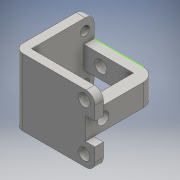
# Autodesk Inventor part: 240510_3Dsketch04
Saved by Autodesk Inventor 2016 (Build 200138000, 138)
## iProperties
Created: 2024-05-10
Part Number: 240510_3Dsketch04
Material: 일반
Document SubType Name: Modeling
Designer: pc
Density: 1 g/cm^3
Appearance: 기본값
Author: pc
Autodesk Inventor part; units mm, degrees
ref_plane "YZ Plane" through (0, 0, 0) normal (1, 0, 0) x (0, 1, 0)
ref_plane "XZ Plane" through (0, 0, 0) normal (0, 1, 0) x (-1, 0, 0)
ref_plane "XY Plane" through (0, 0, 0) normal (0, 0, 1) x (1, 0, 0)
sketch "스케치1" plane through (0, 0, 0) normal (0, 0, 1) x (1, 0, 0)
  line L0 (18.1059, -15.875) -> (-18.1059, -15.875)
  line L1 (-18.1059, -15.875) -> (-18.1059, 15.875)
  line L2 (-18.1059, 15.875) -> (18.1059, 15.875)
  line L3 (18.1059, 15.875) -> (18.1059, -15.875)
  line L4 (18.1059, -15.875) -> (-18.1059, 15.875) construction
  line L5 (-18.1059, -15.875) -> (18.1059, 15.875) construction
  point P0 (0, 0)
  constraints: 12 end point, 2 midpoint, 2 parallel, 1 horizontal, 1 perpendicular
extrude "돌출1" add sketch "스케치1" along normal blind 30
sketch "스케치2" plane through (-18.1059, 15.875, 0) normal (0, 1, 0) x (1, 0, 0)
  line L0 (0, -30) -> (36.2119, -30) projected
  line L1 (36.2119, 0) -> (36.2119, -30) projected
  line L2 (4.0585, -30) -> (36.2119, -30)
  line L3 (36.2119, -30) -> (36.2119, -19.9659)
  line L4 (36.2119, -19.9659) -> (4.0585, -19.9659)
  line L5 (4.0585, -19.9659) -> (4.0585, -30)
  line L6 (36.2119, 0) -> (0, 0) projected
  line L7 (4.0585, 0) -> (36.2119, 0)
  line L8 (36.2119, 0) -> (36.2119, -10.034)
  line L9 (36.2119, -10.034) -> (4.0585, -10.034)
  line L10 (4.0585, -10.034) -> (4.0585, 0)
  point P0 (18.1059, 0)
  dimension "d2" = 10.034
  constraints: 16 end point, 5 point on line, 4 parallel, 2 horizontal, 2 perpendicular
  measures "d2" distance of L7.end L8.end
extrude "돌출2" cut sketch "스케치2" against normal blind 28
sketch "스케치3" plane through (-18.1059, 15.875, 30) normal (0, 1, 0) x (1, 0, 0)
  line L0 (4.0585, 10.0341) -> (36.2119, 10.0341) projected
  line L1 (36.2119, 30) -> (36.2119, 0) projected
  line L2 (31.9669, 10.0341) -> (36.2119, 10.0341)
  line L3 (36.2119, 10.0341) -> (36.2119, 20.0064)
  line L4 (36.2119, 20.0064) -> (31.9669, 20.0064)
  line L5 (31.9669, 20.0064) -> (31.9669, 10.0341)
  point P0 (18.1059, 30)
  constraints: 8 end point, 2 parallel, 2 point on line, 1 horizontal, 1 perpendicular
extrude "돌출3" cut sketch "스케치3" against normal blind 50
sketch "스케치4" plane through (-14.0475, -12.125, 19.9659) normal (0, 0, 1) x (1, 0, 0)
  line L0 (0, 0) -> (22.1415, 0)
  line L1 (22.1415, 0) -> (22.1415, 23.4499)
  line L2 (22.1415, 23.4499) -> (0, 23.4499)
  line L3 (0, 23.4499) -> (0, 0)
  point P0 (14.0475, 12.125)
  constraints: 8 end point, 2 parallel, 1 horizontal, 1 perpendicular
extrude "돌출4" cut sketch "스케치4" against normal blind 50
sketch "스케치5" plane through (-14.0475, 15.875, 30) normal (1, 0, 0) x (0, 0, -1)
  circle A0 centre (5.0001, -4.0724) radius 2.0226
  circle A1 centre (25.7482, -4.0724) radius 2.1705
  point P0 (30, -15.875)
  constraints: 2 centre point
extrude "돌출5" cut sketch "스케치5" against normal blind 50
sketch "스케치6" plane through (-18.1059, -12.125, 0) normal (0, 1, 0) x (1, 0, 0)
  circle A0 centre (31.4326, -4.8571) radius 2.5553
  circle A1 centre (31.4326, -25.7502) radius 2.6688
  point P0 (18.1059, 0)
  constraints: 2 centre point
extrude "돌출6" cut sketch "스케치6" against normal blind 50
sketch "스케치7" plane through (-18.1059, 15.875, 30) normal (0, 1, 0) x (1, 0, 0)
  circle A0 centre (11.6135, 14.7451) radius 2.7078
  point P0 (18.1059, 30)
  constraints: 1 centre point
extrude "돌출7" cut sketch "스케치7" against normal blind 20
sketch "스케치8" plane through (13.861, 15.875, 19.9659) normal (1, 0, 0) x (0, 0, -1)
  circle A0 centre (4.9416, -23.8738) radius 2.5891
  point P0 (19.9659, -15.875)
  constraints: 1 centre point
extrude "돌출8" cut sketch "스케치8" against normal blind 20
fillet "모깎기1" radius 6 1 edges at (13.861, 15.875, 15)
fillet "모깎기2" radius 4 5 edges at (-16.0767, 15.875, 30) (-16.0767, 15.875, 0) (-18.1059, -15.875, 15) (18.1059, -14, 30) (18.1059, -14, 0)
sketch "스케치9" plane through (-14.0475, 15.875, 19.9659) normal (0, 1, 0) x (1, 0, 0)
  line L0 (-4.0585, 15.9659) -> (-4.0585, -6.0341) projected
  line L1 (-4.0585, 9.9335) -> (21.8906, 9.9335)
  line L2 (21.8906, 9.9335) -> (21.8906, -0.0015)
  line L3 (21.8906, -0.0015) -> (-4.0585, -0.0015)
  line L4 (-4.0585, -0.0015) -> (-4.0585, 9.9335)
  point P0 (14.0475, 19.9659)
  constraints: 8 end point, 2 parallel, 1 horizontal, 1 perpendicular, 1 point on line
sketch "스케치10" plane through (-14.0475, 15.875, 19.9659) normal (0, 1, 0) x (1, 0, 0)
  point P0 (14.0475, 19.9659)
